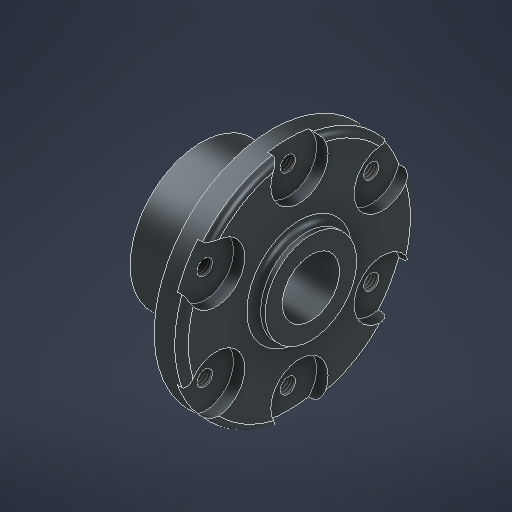
# Autodesk Inventor part: END CAP
Saved by Autodesk Inventor 2026.1 (Build 301233020, 233B)
## iProperties
Created: 2025-10-07
Part Number: END CAP
Material: Iron, Cast
Document SubType Name: Modeling
Designer: elaij
Density: 7.15 g/cm^3
Appearance: Iron Gray
Author: elaij
Autodesk Inventor part; units mm, degrees
ref_plane "YZ Plane" through (0, 0, 0) normal (1, 0, 0) x (0, 1, 0)
ref_plane "XZ Plane" through (0, 0, 0) normal (0, 1, 0) x (-1, 0, 0)
ref_plane "XY Plane" through (0, 0, 0) normal (0, 0, 1) x (1, 0, 0)
sketch "Sketch1" plane through (0, 0, 0) normal (1, 0, 0) x (0, 1, 0)
  circle A0 centre (0, 0) radius 51.5
  circle A1 centre (0, 0) radius 31
  circle A2 centre (0, 0) radius 11
  dimension "d0" = 103
  dimension "d2" = 62
  dimension "d3" = 22
  constraints: 3 centre point, 3 coincident
  measures "d0" diameter of A0
  measures "d2" diameter of A1
  measures "d3" diameter of A2
extrude "Extrusion1" add sketch "Sketch1" along normal blind 12 contours A0 | A1 | A2
sketch "Sketch3" plane through (0, 0, 0) normal (-1, 0, 0) x (0, 0, 1)
  circle A0 centre (0, 0) radius 11 projected
  circle A1 centre (0, 0) radius 31
  dimension "d13" = 62
  constraints: 1 centre point, 1 coincident
  measures "d13" diameter of A1
extrude "Extrusion2" add sketch "Sketch3" along normal blind 60 contours A0 | A1
sketch "Sketch4" plane through (12, 0, 0) normal (1, 0, 0) x (0, 0, -1)
  circle A0 centre (0, 0) radius 20
  dimension "d16" = 40
  constraints: 1 centre point, 1 coincident
  measures "d16" diameter of A0
extrude "Extrusion3" add sketch "Sketch4" along normal blind 5
sketch "Sketch6" plane through (12, 0, 0) normal (1, 0, 0) x (0, 0, -1)
  circle A0 centre (0, 0) radius 11 projected
  circle A1 centre (0, 0) radius 42
  line L0 (0, 0) -> (0, 42)
  point P0 (0.0095, 11)
  point P1 (0.0095, -11)
  point P2 (-36.3731, 21)
  point P3 (-36.3731, -21)
  point P4 (0, -42)
  point P5 (36.3731, -21)
  point P6 (36.3731, 21)
  dimension "d30" = 84
  dimension "d28" = 360
  constraints: 2 coincident, 2 end point, 1 vertical, 1 vertical alignment, 9 other
hole "Hole3" at (12, 42, 0) at (12, 21, 36.3731) at (12, -21, 36.3731) at (12, -42, 0) at (12, -21, -36.3731) at (12, 21, -36.3731) direction (-1, 0, 0) diameter 6.647 end through all counterbore diameter 25 counterbore depth 5 thread size "M8x1.25" class "6H" standard "ISO Metric profile"
thread "Thread1" size "M8x1.25" class "6H" standard "ANSI Metric M Profile" full length
sketch "Sketch7" plane through (17, 0, 0) normal (1, 0, 0) x (0, 0, -1)
  circle A0 centre (0, 0) radius 20 projected
  circle A1 centre (0, 0) radius 12.5
  dimension "d40" = 25
  constraints: 1 centre point, 1 coincident
  measures "d40" diameter of A1
extrude "Extrusion4" cut sketch "Sketch7" against normal blind 100 contours A1
fillet "Fillet1" radius 3 6 edges at (12, 44.6003, 25.75) (12, 0, 51.5) (12, -44.6003, 25.75) (12, -44.6003, -25.75) (12, 0, -51.5) (12, 44.6003, -25.75)
fillet "Fillet2" radius 3 1 edges at (12, 0, 20)
sketch "Sketch8" plane through (-60, 0, 0) normal (-1, 0, 0) x (0, 0, 1)
  circle A0 centre (0, 0) radius 23.5
  dimension "d45" = 47
  constraints: 1 centre point, 1 coincident
  measures "d45" diameter of A0
extrude "Extrusion5" cut sketch "Sketch8" against normal blind 55
sketch "Sketch9" plane through (-60, 0, 0) normal (-1, 0, 0) x (0, 0, 1)
  circle A0 centre (0, 0) radius 11 projected
  circle A1 centre (0, 0) radius 31
  circle A2 centre (0, 0) radius 31 projected
  constraints: 1 centre point, 1 coincident, 1 concentric
extrude "Extrusion6" cut sketch "Sketch9" against normal blind 29 contours A0 | A1
chamfer "Chamfer1" distance 5 angle 15 1 edges at (-31, 0, -23.5) measured on face at (-30.5, 0, -23.5)
body "Solid1"
